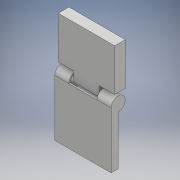
# Autodesk Inventor part: hinge
Saved by Autodesk Inventor 2018.2 (Build 222227000, 227)
## iProperties
Created: 2018-03-24
Part Number: hinge
Material: Generic
Document SubType Name: Modeling
Designer: wharr
Density: 1 g/cm^3
Appearance: Default
Author: wharr
Autodesk Inventor part; units mm, degrees
ref_plane "YZ Plane" through (0, 0, 0) normal (1, 0, 0) x (0, 1, 0)
ref_plane "XZ Plane" through (0, 0, 0) normal (0, 1, 0) x (-1, 0, 0)
ref_plane "XY Plane" through (0, 0, 0) normal (0, 0, 1) x (1, 0, 0)
sketch "Sketch1" plane through (0, 0, 0) normal (0, 1, 0) x (-1, 0, 0)
  line L0 (-12.7, 12.7) -> (12.7, 12.7)
  line L1 (12.7, 12.7) -> (12.7, -12.7)
  line L2 (12.7, -12.7) -> (-12.7, -12.7)
  line L3 (-12.7, -12.7) -> (-12.7, 12.7)
  line L4 (-12.7, 12.7) -> (12.7, -12.7) construction
  line L5 (12.7, 12.7) -> (-12.7, -12.7) construction
  point P0 (0, 0)
  dimension "d0" = 25.4
  dimension "d1" = 25.4
  constraints: 12 end point, 2 midpoint, 2 parallel, 1 horizontal, 1 perpendicular
  measures "d0" distance of L1.end L2.end
  measures "d1" distance of L0.end L1.end
extrude "Extrusion1" add sketch "Sketch1" along normal blind 3.175
sketch "Sketch2" plane through (12.7, 0, 12.7) normal (1, 0, 0) x (0, 0, -1)
  circle A0 centre (0, 3.175) radius 3.175
  point P0 (12.7, 0)
  constraints: 1 centre point
extrude "Extrusion2" add sketch "Sketch2" against normal blind 6.35
mirror "Mirror1" about plane through (0, 0, 0) normal (1, 0, 0) of "Extrusion2"
sketch "Sketch3" plane through (6.35, 0, 12.7) normal (-1, 0, 0) x (0, 0, 1)
  arc A0 (0, 0) -> (-3.175, 3.175) centre (0, 3.175) ccw projected
  circle A1 centre (0, 3.175) radius 2.54
  point P0 (-12.7, 0)
  dimension "d6" = 0.635
  constraints: 1 centre point, 1 coincident
  measures "d6" radial gap between concentric circles of A1 A0
extrude "Extrusion3" cut sketch "Sketch3" against normal blind 4.7625 and the other way blind 17.4625
ref_plane "Work Plane1" through (-9.525, 3.175, 12.7) normal (1, 0, 0) x (0, 0, -1)
ref_plane "Work Plane2" through (9.525, 3.175, 12.7) normal (-1, 0, 0) x (0, 0, 1)
sketch "Sketch5" plane through (9.525, 3.175, 12.7) normal (-1, 0, 0) x (0, 0, 1)
  arc A0 (0, -2.54) -> (-2.54, 0) centre (0, 0) ccw projected
  circle A1 centre (0, 0) radius 1.5875
  point P0 (-12.7, -3.175)
  dimension "d13" = 3.175
  constraints: 1 centre point, 1 coincident
  measures "d13" diameter of A1
extrude "Extrusion4" add sketch "Sketch5" along normal up to surface (19.05 mm away)
sketch "Sketch6" plane through (0, 0, 0) normal (1, 0, 0) x (0, 1, 0)
  circle A0 centre (3.175, 12.7) radius 1.5875 projected
  circle A1 centre (3.175, 12.7) radius 1.5875 projected
  arc A2 (1.5875, 12.7) -> (4.7625, 12.7) centre (3.175, 12.7) ccw
  line L0 (1.5875, 12.7) -> (1.5875, 17.145)
  circle A3 centre (3.175, 12.7) radius 1.5875 projected
  line L1 (4.7625, 17.145) -> (4.7625, 12.7)
  arc A4 (3.175, 9.525) -> (0, 12.7) centre (3.175, 12.7) ccw projected
  line L2 (1.5875, 17.145) -> (4.7625, 17.145)
  line L3 (1.5875, 15.875) -> (4.7625, 15.875) construction
  point P0 (0, 0)
  dimension "d18" = 1.27
  constraints: 8 end point, 5 tangent, 2 point on circle, 2 point on line, 2 vertical, 1 centre point, 1 coincident, 1 concentric, 1 horizontal, 1 horizontal alignment, 1 parallel, 1 perpendicular
  measures "d18" distance between parallel lines of L2 L3
extrude "Extrusion5" add sketch "Sketch6" along normal mid plane 11.43 contours A0 L0 A4 L1 | A4 L0 L2 L1
sketch "Sketch9" plane through (-5.715, 1.5875, 12.7) normal (0, -1, 0) x (1, 0, 0)
  line L0 (-6.985, 23.495) -> (18.415, 23.495)
  line L1 (18.415, 23.495) -> (18.415, 4.445)
  line L2 (18.415, 4.445) -> (-6.985, 4.445)
  line L3 (-6.985, 4.445) -> (-6.985, 23.495)
  line L4 (0, 4.445) -> (11.43, 4.445) projected
  line L5 (18.415, -25.4) -> (18.415, 0) projected
  point P0 (5.715, -12.7)
  dimension "d25" = 25.4
  dimension "d26" = 19.05
  constraints: 8 end point, 2 collinear, 2 parallel, 1 horizontal, 1 perpendicular
  measures "d25" distance of L1.end L2.end
  measures "d26" distance of L0.end L1.end
extrude "Extrusion8" add sketch "Sketch9" against normal blind 4.7752
body "Solid1"
